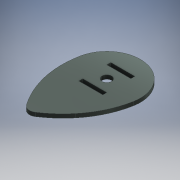
# Autodesk Inventor part: leva00
Saved by Autodesk Inventor 2016 (Build 200138000, 138)
## iProperties
Created: 2016-09-20
Part Number: leva00
Material: Madera (abedul)
Document SubType Name: Modeling
Designer: i95sa
Density: 0.55 g/cm^3
Appearance: Gris plomo - Pulido
Author: i95sa
Autodesk Inventor part; units mm, degrees
ref_plane "YZ Plane" through (0, 0, 0) normal (1, 0, 0) x (0, 1, 0)
ref_plane "XZ Plane" through (0, 0, 0) normal (0, 1, 0) x (-1, 0, 0)
ref_plane "XY Plane" through (0, 0, 0) normal (0, 0, 1) x (1, 0, 0)
sketch "Boceto1" plane through (0, 0, 0) normal (0, 0, 1) x (1, 0, 0)
  arc A0 (6.5527, 34.3506) -> (-6.5527, -34.3506) centre (0, 0) ccw
  arc A1 (-10.0841, -52.8628) -> (-13.1085, -68.717) centre (-11.5963, -60.7899) ccw
  line L0 (-13.5463, -71.0121) -> (-21.4733, -69.4999)
  line L1 (-34.2706, 6.9592) -> (-47.4823, 9.4795)
  line L2 (-47.4823, 9.4795) -> (-21.4733, -69.4999)
  line L3 (-21.4733, -69.4999) -> (-31.5702, -38.8396)
  arc A2 (-34.2706, 6.9592) -> (-31.5702, -38.8396) centre (53.4264, -10.8491) ccw
  arc A3 (-31.5702, -38.8396) -> (-18.1931, -65.4383) centre (64.4102, -7.232) ccw
  line L4 (0.5041, 2.6424) -> (6.5527, 34.3506)
  line L5 (-0.5041, -2.6424) -> (-13.5463, -71.0121)
  arc A4 (-6.5527, -34.3506) -> (6.5527, 34.3506) centre (0, 0) ccw
  arc A5 (-13.1085, -68.717) -> (-10.0841, -52.8628) centre (-11.5963, -60.7899) ccw
  line L6 (-13.5463, -71.0121) -> (-5.6192, -72.5242)
  line L7 (34.4258, -6.1454) -> (47.6376, -8.6656)
  line L8 (47.6376, -8.6656) -> (-5.6192, -72.5242)
  line L9 (-5.6192, -72.5242) -> (15.0554, -47.7339)
  arc A6 (15.0554, -47.7339) -> (34.4258, -6.1454) centre (-53.6684, 9.5804) ccw
  arc A7 (-7.174, -67.5403) -> (15.0554, -47.7339) centre (-62.5493, 16.9869) ccw
  dimension "d0" = 69.94
  dimension "d6" = 16.14
  dimension "d7" = 8.07
  dimension "d8" = 13.45
  dimension "d9" = 32.28
  constraints: 20 end point, 20 point on circle, 8 centre point, 6 symmetric about line, 5 point on line, 4 tangent, 1 collinear, 4 other
  measures "d0" diameter of A0
  measures "d6" diameter of A1
  measures "d7" distance of L0.start L0.end
  measures "d8" distance of L1.start L1.end
  measures "d9" distance of L0.end L3.end
extrude "Extrusión2" add sketch "Boceto1" along normal blind 4 contours A4 A0 | A0 L5 A1 A3 A2 | A6 A7 A5 L5 A4 | L5 A1 | A5 L5
sketch "Boceto2" plane through (0, 0, 4) normal (0, 0, 1) x (1, 0, 0)
  line L0 (0, 0) -> (0, 12.5)
  line L1 (0, 12.5) -> (-12.5, 12.5)
  line L2 (-12.5, 12.5) -> (-12.5, 16.7)
  line L3 (-12.5, 16.7) -> (12.5, 16.7)
  line L4 (12.5, 16.7) -> (12.5, 12.5)
  line L5 (12.5, 12.5) -> (0, 12.5)
  line L6 (0, 0) -> (12.5, 0)
  line L7 (0, 0) -> (0, -12.5)
  line L8 (0, -12.5) -> (-12.5, -12.5)
  line L9 (-12.5, -12.5) -> (-12.5, -16.7)
  line L10 (-12.5, -16.7) -> (12.5, -16.7)
  line L11 (12.5, -16.7) -> (12.5, -12.5)
  line L12 (12.5, -12.5) -> (0, -12.5)
  circle A0 centre (0, 0) radius 5
  dimension "d24" = 12.5
  dimension "d25" = 12.5
  dimension "d26" = 4.2
  dimension "d27" = 25
  dimension "d28" = 10
  constraints: 26 end point, 5 perpendicular, 5 symmetric about line, 3 point on line, 1 centre point, 1 coincident, 1 parallel, 1 vertical
  measures "d24" distance of L0.start L0.end
  measures "d25" distance of L0.end L1.end
  measures "d26" distance of L1.end L2.end
  measures "d27" distance of L2.end L3.end
  measures "d28" diameter of A0
extrude "Extrusión3" cut sketch "Boceto2" against normal blind 4
